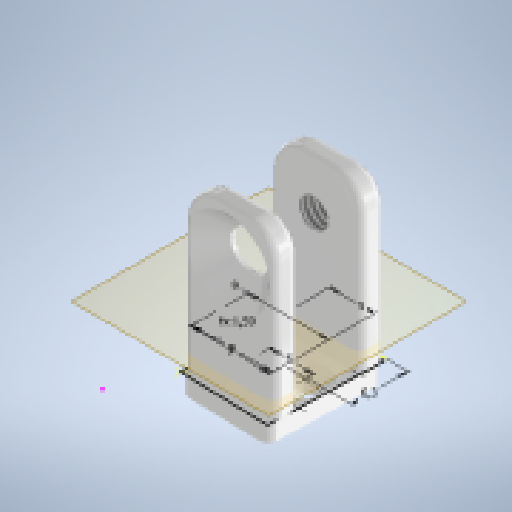
# Autodesk Inventor part: HalterUmlenkrolleOVR
Saved by Autodesk Inventor 2025 (Build 290162010, 162A)
## iProperties
Created: 2024-11-18
Part Number: HalterUmlenkrolleOVR
Material: PC/ABS-Kunststoff, 3DDruck, PLA
Document SubType Name: Modeling
Designer: Admin
Density: 1.1 g/cm^3
Appearance: Glatt - Weiß(2)
Mass: 1.27265 g
Surface Area: 12.7122 cm^2
Volume: 1.15695 cm^3
Author: Admin
Autodesk Inventor part; units mm, degrees
note: some values were not read from the file. Chosen so that the rebuilt part matches the saved one: direction of "Bohrung1".
ref_plane "YZ Plane" through (0, 0, 0) normal (1, 0, 0) x (0, 1, 0)
ref_plane "XZ Plane" through (0, 0, 0) normal (0, 1, 0) x (-1, 0, 0)
ref_plane "XY Plane" through (0, 0, 0) normal (0, 0, 1) x (1, 0, 0)
sketch "Skizze1" plane through (0, 0, 0) normal (0, 0, 1) x (1, 0, 0)
  line L0 (12.8939, 18.6723) -> (2.8939, 18.6723)
  line L1 (2.8939, 18.6723) -> (2.8939, 15.6723)
  line L2 (2.8939, 15.6723) -> (12.8939, 15.6723)
  line L3 (12.8939, 15.6723) -> (12.8939, 18.6723)
  line L4 (12.8939, 9.0723) -> (2.8939, 9.0723)
  line L5 (2.8939, 9.0723) -> (2.8939, 6.0723)
  line L6 (2.8939, 6.0723) -> (12.8939, 6.0723)
  line L7 (12.8939, 6.0723) -> (12.8939, 9.0723)
  line L8 (12.8939, 15.6723) -> (12.8939, 12.3723) construction
  line L9 (12.8939, 12.3723) -> (12.8939, 9.0723) construction
  point P0 (0, 0)
  point P1 (7.8939, 9.0723)
  dimension "d0" = 10
  dimension "d1" = 3
  dimension "d2" = 3
  dimension "d3" = 6.6
  constraints: 20 end point, 5 equal length, 3 horizontal, 2 collinear, 2 perpendicular, 2 vertical, 1 midpoint
  measures "d0" distance of L2.end L1.end
  measures "d1" distance of L0.end L1.end
  measures "d2" distance of L4.end L5.end
  measures "d3" distance from line of point (7.894, 9.072) L2
extrude "Extrusion1" add sketch "Skizze1" along normal blind 18
fillet "Rundung1" radius 3 4 edges at (12.8939, 7.5723, 18) (12.8939, 17.1723, 18) (2.8939, 17.1723, 18) (2.8939, 7.5723, 18)
sketch "Skizze2" plane through (2.8939, 6.0723, 0) normal (0, -1, 0) x (1, 0, 0)
  circle A0 centre (5, 13) radius 5 construction
  line L0 (10, 0) -> (10, 15) construction
  line L1 (0, 0) -> (0, 15) construction
  line L2 (3, 18) -> (7, 18) construction
  point P0 (-2.8939, 0)
  constraints: 3 tangent, 1 centre point
hole "Bohrung1" at (7.8939, 6.0723, 13) direction (0, 1, 0) diameter 4.3 depth 3 countersink diameter 9.4 countersink angle 90 clearance for "Flachkopfmaschinenschraube" size "M4" standard "ANSI Metrisches M Profil"
ref_plane "Arbeitsebene1" through (2.8939, 15.6723, 2) normal (0, 0, 1) x (1, 0, 0)
sketch "Skizze4" plane through (2.8939, 15.6723, 0) normal (0, 0, 1) x (1, 0, 0)
  line L0 (10, -3.3) -> (10, 0) construction
  line L1 (10, -3.3) -> (10, -6.6) construction
  line L2 (0, -3.3) -> (0, -6.6) construction
  line L3 (0, 0) -> (0, -3.3) construction
  line L4 (10, 3) -> (0, 3) construction
  line L5 (0, 3) -> (0, 0) construction
  line L6 (-4, -3.3) -> (5, -3.3) construction
  line L7 (-4, -3.3) -> (4.9965, -3.5494) construction
  line L8 (-4, -3.3) -> (5, -3.3) construction
  line L9 (2.4975, -3.4801) -> (4.9965, -3.5494) construction
  line L10 (4.9965, -3.5494) -> (7.4956, -3.6186) construction
  line L11 (0, 3) -> (0, 0) projected
  line L12 (10, 3) -> (0, 3) projected
  line L13 (-0.1761, -9.7084) -> (9.8201, -9.9855)
  line L14 (9.8201, -9.9855) -> (10.1692, 2.6097)
  line L15 (10.1692, 2.6097) -> (0.173, 2.8868)
  line L16 (0.173, 2.8868) -> (-0.1761, -9.7084)
  line L17 (0, 3) -> (0, -9.6) construction
  line L18 (9.9946, -3.6879) -> (4.9965, -3.5494) construction
  line L19 (4.9965, -3.5494) -> (-0.0015, -3.4108) construction
  point P0 (-2.8939, -15.6723)
  dimension "d34" = 5
  dimension "d35" = 9
  dimension "d36" = 6.3
  dimension "d37" = 5
  dimension "d38" = 9
  dimension "d40" = 9
  dimension "d41" = 1.588
  constraints: 36 end point, 7 equal length, 6 collinear, 5 coincident, 3 vertical, 2 midpoint, 2 parallel, 2 perpendicular, 1 horizontal, 1 point on line
  measures "d34" distance of L9.start L10.end
  measures "d35" distance of L6.start point (5, -3.3)
  measures "d36" distance from line of L4 point (5, -3.3)
  measures "d37" distance from line of L5 point (5, -3.3)
  measures "d38" distance of L6.start L6.end
  measures "d40" distance of L6.start L7.end
  measures "d41" angle of L7 L8
extrude "Extrusion3" add sketch "Skizze4" against normal blind 2
hole "Bohrung2" at (10.3894, 12.0537, 0) at (5.3914, 12.1923, 0) direction (0, 0, -1) diameter 2 end through all countersink diameter 5 countersink angle 90
sketch "Skizze5" plane through (2.8939, 6.0723, 0) normal (0, -1, 0) x (1, 0, 0)
  circle A0 centre (5, 13) radius 4.7 projected
  point P0 (-2.8939, 0)
hole "Bohrung3" at (7.8939, 6.0723, 13) direction (0, 1, 0) diameter 3.242 end through all thread size "M4x0.7" class "6H" standard "ANSI Metric M Profile"
fillet "Rundung2" radius 1 23 edges at (3.7725, 6.0723, 17.1213) (7.8939, 6.0723, 18) (12.0152, 6.0723, 17.1213) (12.8939, 6.0723, 7.5) (2.8939, 6.0723, 7.5) (3.7725, 9.0723, 17.1213) (7.8939, 9.0723, 18) (12.0152, 9.0723, 17.1213) (12.8939, 9.0723, 7.5) (2.8939, 9.0723, 7.5) (7.8939, 15.6723, 18) (12.0152, 15.6723, 17.1213) (12.8939, 15.6723, 7.5) (2.8939, 15.6723, 7.5) (3.7725, 15.6723, 17.1213) (2.8939, 18.6723, 7.5) (7.8939, 18.6723, 18) (12.0152, 18.6723, 17.1213) (12.8939, 18.6723, 7.5) (3.7725, 18.6723, 17.1213) (2.7178, 5.9639, -1) (12.7139, 5.6869, -1) (13.063, 18.282, -1)
equation "\"d41\" = schrägWinkel"
equation "\"schrägWinkel\" = 1.587669deg"
